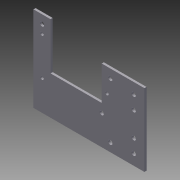
# Autodesk Inventor part: AS5-8-5-001
Saved by Autodesk Inventor 2011 SP1 (Build 150282100, 282)
## iProperties
Created: 2011-01-12
Part Number: AS5-8-5-001
Document SubType Name: Modeling
Designer: Christopher
Density: 1 g/cm^3
Author: Christopher
Autodesk Inventor part; units mm, degrees
ref_plane "YZ Plane" through (0, 0, 0) normal (1, 0, 0) x (0, 1, 0)
ref_plane "XZ Plane" through (0, 0, 0) normal (0, 1, 0) x (-1, 0, 0)
ref_plane "XY Plane" through (0, 0, 0) normal (0, 0, 1) x (1, 0, 0)
sketch "Sketch1" plane through (0, 0, 0) normal (0, 0, 1) x (1, 0, 0)
  line L0 (106.0233, -22.2944) -> (-20.9767, -22.2944)
  line L1 (-20.9767, -22.2944) -> (-20.9767, 104.7056)
  line L2 (4.4233, 104.7056) -> (4.4233, 34.8556)
  line L3 (4.4233, 34.8556) -> (80.6233, 34.8556)
  line L4 (-20.9767, 104.7056) -> (4.4233, 104.7056)
  line L5 (106.0233, -22.2944) -> (106.0233, 85.6556)
  line L6 (106.0233, 85.6556) -> (80.6233, 85.6556)
  line L7 (80.6233, 85.6556) -> (80.6233, 34.8556)
  line L8 (106.0233, 85.6556) -> (144.1233, 85.6556)
  line L9 (144.1233, 85.6556) -> (144.1233, -22.2944)
  line L10 (144.1233, -22.2944) -> (106.0233, -22.2944)
  point P0 (0, 0)
  point P1 (-8.2767, 79.4563)
  point P2 (-8.2767, 22.6873)
  point P3 (88.3779, 51.0718)
  point P4 (93.3233, 72.9556)
  point P5 (-8.2767, 92.0056)
  point P6 (80.6233, 22.1556)
  point P7 (93.3233, -9.5944)
  point P8 (128.2483, 13.5704)
  point P9 (128.2483, -6.4194)
  point P10 (128.2483, 69.7552)
  point P11 (128.2483, 49.7654)
  dimension "d0" = 127
  dimension "d5" = 56.769
  dimension "d6" = 96.6546
  dimension "d7" = 12.7
  dimension "d8" = 25.4
  dimension "d9" = 76.2
  dimension "d12" = 107.95
  dimension "d13" = 25.4
  dimension "d14" = 50.8
  dimension "d22" = 28.3845
  dimension "d23" = 127
  dimension "d24" = 25.4
  dimension "d25" = 12.7
  dimension "d26" = 12.7
  dimension "d27" = 44.45
  dimension "d29" = 12.7
  dimension "d30" = 12.7
  dimension "d38" = 12.7
  dimension "d39" = 12.7
  dimension "d40" = 38.1
  dimension "d41" = 107.95
  dimension "d42" = 19.9898
  dimension "d43" = 15.875
  dimension "d53" = 15.875
  dimension "d54" = 15.875
  dimension "d55" = 15.875
  dimension "d56" = 15.875
  dimension "d57" = 15.9004
  dimension "d58" = 19.9898
  constraints: 22 end point, 7 perpendicular, 3 parallel, 1 point on line
  measures "d0" distance of L0.end L1.end
  measures "d5" distance of point (-8.277, 22.687) point (-8.277, 79.456)
  measures "d6" horizontal distance of point (-8.277, 79.456) point (88.378, 51.072)
  measures "d7" distance from line of L1 point (-8.277, 79.456)
  measures "d8" distance of L1.end L2.start
  measures "d9" distance of L2.end L3.end
  measures "d12" distance of L0.start L5.end
  measures "d13" distance of L5.end L6.end
  measures "d14" distance of L6.end L3.end
  measures "d22" vertical distance of point (-8.277, 79.456) point (88.378, 51.072)
  measures "d23" distance of L0.start L0.end
  measures "d24" distance from line of L5 point (80.623, 22.156)
  measures "d25" distance from line of L5 point (93.323, 72.956)
  measures "d26" distance from line of L6 point (93.323, 72.956)
  measures "d27" distance from line of L0 point (80.623, 22.156)
  measures "d29" distance from line of L1 point (-8.277, 92.006)
  measures "d30" distance from line of point (-8.277, 92.006) L4
  measures "d38" distance from line of L5 point (93.323, -9.594)
  measures "d39" distance from line of L0 point (93.323, -9.594)
  measures "d40" distance of L9.end L0.start
  measures "d41" distance of L8.end L9.end
  measures "d42" distance of point (128.248, 13.57) point (128.248, -6.419)
  measures "d43" distance from line of L10 point (128.248, -6.419)
  measures "d53" distance from line of L9 point (128.248, -6.419)
  measures "d54" distance from line of L9 point (128.248, 13.57)
  measures "d55" distance from line of L9 point (128.248, 49.765)
  measures "d56" distance from line of L9 point (128.248, 69.755)
  measures "d57" distance from line of L8 point (128.248, 69.755)
  measures "d58" distance of point (128.248, 69.755) point (128.248, 49.765)
extrude "Extrusion1" add sketch "Sketch1" against normal blind 3.175 contours L0 L1 L4 L2 L3 L7 L6 L5
hole "Hole1" at (-8.2767, 79.4563, 0) at (-8.2767, 22.6873, 0) at (88.3779, 51.0718, 0) direction (0, 0, -1) diameter 5.0038 depth 25.4 tip angle 118
hole "Hole2" at (93.3233, 72.9556, 0) at (-8.2767, 92.0056, 0) at (80.6233, 22.1556, 0) at (93.3233, -9.5944, 0) direction (0, 0, -1) diameter 6.35 depth 25.4 tip angle 118
extrude "Extrusion2" add sketch "Sketch1" against normal blind 3.175 contours L5 L8 L9 L10
hole "Hole3" at (128.2483, 13.5704, 0) at (128.2483, -6.4194, 0) at (128.2483, 69.7552, 0) at (128.2483, 49.7654, 0) direction (0, 0, -1) diameter 6.35 depth 25.4 tip angle 118
body "Solid1"
